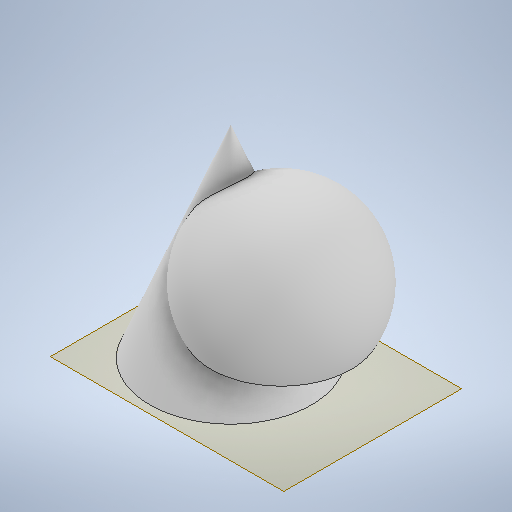
# Autodesk Inventor part: Деталь2
Saved by Autodesk Inventor 2025 (Build 290162000, 162)
## iProperties
Created: 2024-11-19
Part Number: Деталь2
Material: Типовые
Document SubType Name: Modeling
Designer: shoptick
Density: 1 g/cm^3
Appearance: По умолчанию
Author: shoptick
Autodesk Inventor part; units mm, degrees
ref_plane "YZ Plane" through (0, 0, 0) normal (1, 0, 0) x (0, 1, 0)
ref_plane "XY Plane" through (0, 0, 0) normal (0, 0, 1) x (1, 0, 0)
sketch "Эскиз1" plane through (0, 0, 0) normal (0, 0, 1) x (1, 0, 0)
  line L0 (0, 0) -> (-40, 0)
  line L1 (0, 0) -> (0, 100)
  line L2 (0, 100) -> (-40, 0)
  dimension "d0" = 40
  dimension "d1" = 100
  constraints: 6 end point, 1 horizontal, 1 vertical
  measures "d0" distance of L0.start L0.end
  measures "d1" distance of L0.start L1.end
revolve "Вращение1" add sketch "Эскиз1" angle 360 about axis through (0, 0, 0) along (0, 1, 0)
sketch "Эскиз2" plane through (0, 0, 0) normal (0, 0, 1) x (1, 0, 0)
  line L0 (40, 0) -> (-40, 0) projected
  arc A0 (59.641, 25) -> (25, 85) centre (25, 45) ccw
  line L1 (25, 25) -> (25, 85)
  line L2 (25, 25) -> (59.641, 25)
  point P0 (0, 0)
  dimension "d5" = 80
  constraints: 4 end point, 2 point on circle, 1 centre point, 1 horizontal, 1 vertical
  measures "d5" diameter of A0
revolve "Вращение2" add sketch "Эскиз2" angle 360 about axis through (25, 25, 0) along (0, 1, 0)
